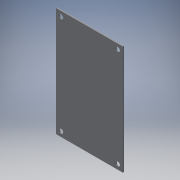
# Autodesk Inventor part: PCBBase
Saved by Autodesk Inventor 2016 (Build 200138000, 138)
## iProperties
Created: 2018-10-10
Part Number: PCBBase
Material: Generic
Document SubType Name: Modeling
Designer: vtolenti89
Density: 1 g/cm^3
Appearance: LED - Green Off
Author: vtolenti89
Autodesk Inventor part; units mm, degrees
ref_plane "YZ Plane" through (0, 0, 0) normal (1, 0, 0) x (0, 1, 0)
ref_plane "XZ Plane" through (0, 0, 0) normal (0, 1, 0) x (-1, 0, 0)
ref_plane "XY Plane" through (0, 0, 0) normal (0, 0, 1) x (1, 0, 0)
sketch "Sketch1" plane through (0, 0, 0) normal (0, 0, 1) x (1, 0, 0)
  line L0 (-85, 9) -> (5, 9) construction
  line L1 (9, 5) -> (9, -145) construction
  line L2 (-89, -145) -> (-89, 5) construction
  circle A0 centre (0, -140) radius 6 construction
  circle A1 centre (0, 0) radius 6 construction
  circle A2 centre (-80, 0) radius 6 construction
  circle A3 centre (-80, -140) radius 6 construction
  arc A4 (-89, -145) -> (-85, -149) centre (-85, -145) ccw construction
  line L3 (5, -149) -> (-85, -149) construction
  arc A5 (5, -149) -> (9, -145) centre (5, -145) ccw construction
  line L4 (9, 5) -> (9, -145) construction
  arc A6 (9, 5) -> (5, 9) centre (5, 5) ccw construction
  line L5 (-85, 9) -> (5, 9) construction
  arc A7 (-85, 9) -> (-89, 5) centre (-85, 5) ccw construction
  line L6 (-89, -145) -> (-89, 5) construction
  circle A8 centre (0, 0) radius 2.5 construction
  circle A9 centre (0, -140) radius 2.5 construction
  circle A10 centre (-80, -140) radius 2.5 construction
  circle A11 centre (-80, 0) radius 2.5 construction
  circle A12 centre (0, 0) radius 3
  circle A13 centre (0, -140) radius 3
  circle A14 centre (-80, -140) radius 3
  circle A15 centre (-80, 0) radius 3
  line L7 (7, 7) -> (-87, 7)
  line L8 (-87, 7) -> (-87, -147)
  line L9 (-87, -147) -> (7, -147)
  line L10 (7, -147) -> (7, 7)
  point P0 (0, 0)
  dimension "d0" = 6
  dimension "d1" = 6
  dimension "d2" = 6
  dimension "d3" = 6
  dimension "d4" = 7
  dimension "d5" = 7
  dimension "d6" = 7
  dimension "d7" = 7
  constraints: 8 end point, 4 centre point, 4 coincident, 2 parallel, 1 horizontal, 1 perpendicular
  measures "d0" diameter of A12
  measures "d1" diameter of A13
  measures "d2" diameter of A14
  measures "d3" diameter of A15
  measures "d4" distance from line of L9 A3.centre
  measures "d5" distance from line of A3.centre L8
  measures "d6" distance from line of A0.centre L10
  measures "d7" distance from line of A1.centre L7
extrude "Extrusion1" add sketch "Sketch1" along normal blind 1.6
body "Solid1"
